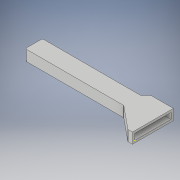
# Autodesk Inventor part: PATAS
Saved by Autodesk Inventor 2019 (Build 230136000, 136)
## iProperties
Created: 2020-12-04
Part Number: PATAS
Material: Generic
Document SubType Name: Modeling
Designer: mihai
Density: 1 g/cm^3
Appearance: Default
Author: mihai
Autodesk Inventor part; units mm, degrees
ref_plane "YZ Plane" through (0, 0, 0) normal (1, 0, 0) x (0, 1, 0)
ref_plane "XZ Plane" through (0, 0, 0) normal (0, 1, 0) x (-1, 0, 0)
ref_plane "XY Plane" through (0, 0, 0) normal (0, 0, 1) x (1, 0, 0)
sketch "Sketch1" plane through (0, 0, 0) normal (0, 1, 0) x (-1, 0, 0)
  line L0 (0, 0) -> (0, -48)
  line L1 (0, 0) -> (4.9, 0)
  line L2 (0, -24) -> (33, -24) construction
  line L3 (0, -48) -> (33, -48) construction
  line L4 (33, -48) -> (33, -43) construction
  line L5 (33, -48) -> (28, -48) construction
  line L6 (0, -48) -> (28, -48)
  line L7 (28, -48) -> (33, -43)
  line L8 (33, -43) -> (33, -23)
  line L9 (4.9, 0) -> (33, -23)
  dimension "d0" = 48
  dimension "d1" = 4.9
  dimension "d2" = 33
  dimension "d3" = 5
  dimension "d4" = 5
  dimension "d5" = 20
  constraints: 20 end point, 3 horizontal, 2 vertical, 1 collinear, 1 midpoint, 1 perpendicular, 1 point on line
  measures "d0" distance of L0.start L0.end
  measures "d1" distance of L0.start L1.end
  measures "d2" distance of L2.start L2.end
  measures "d3" distance of L3.end L4.end
  measures "d4" distance of L3.end L5.end
  measures "d5" distance of L4.end L8.end
extrude "Extrusion1" add sketch "Sketch1" along normal blind 1
sketch "Sketch2" plane through (0, 1, 0) normal (0, 1, 0) x (1, 0, 0)
  line L0 (0, 0) -> (0, 48) projected
  line L1 (0, 48) -> (-28, 48) projected
  line L2 (-28, 48) -> (-33, 43) projected
  line L3 (-33, 43) -> (-33, 23) projected
  line L4 (-33, 23) -> (-4.9, 0) projected
  line L5 (-4.9, 0) -> (0, 0) projected
  line L6 (-5.9712, -3) -> (-36, 21.5787)
  line L7 (-36, 21.5787) -> (-36, 44.2426)
  line L8 (-36, 44.2426) -> (-29.2426, 51)
  line L9 (-29.2426, 51) -> (3, 51)
  line L10 (3, 51) -> (3, -3)
  line L11 (3, -3) -> (-5.9712, -3)
  dimension "d8" = 3
  constraints: 12 end point, 5 other
  measures "d8" distance between parallel lines of L4 L6
extrude "Extrusion2" add sketch "Sketch2" along normal blind 3 contours L5 L4 L3 L2 L1 L0 | L6 L7 L8 L9 L10 L11
sketch "Sketch3" plane through (0, 0, 0) normal (0, -1, 0) x (1, 0, 0)
  line L0 (0, 0) -> (0, -48) projected
  line L1 (-4.9, 0) -> (0, 0) projected
  line L2 (-33, -23) -> (-4.9, 0) projected
  line L3 (-33, -43) -> (-33, -23) projected
  line L4 (-28, -48) -> (-33, -43) projected
  line L5 (0, -48) -> (-28, -48) projected
  line L6 (3, -51) -> (3, 3)
  line L7 (3, 3) -> (-5.9712, 3)
  line L8 (-5.9712, 3) -> (-36, -21.5787)
  line L9 (-36, -21.5787) -> (-36, -44.2426)
  line L10 (-36, -44.2426) -> (-29.2426, -51)
  line L11 (-29.2426, -51) -> (3, -51)
  dimension "d11" = 3
  constraints: 12 end point, 5 other
  measures "d11" distance between parallel lines of L0 L6
extrude "Extrusion3" add sketch "Sketch3" along normal blind 3 contours L0 L5 L4 L3 L2 L1 | L11 L10 L9 L8 L7 L6
sketch "Sketch4" plane through (0, 0, 0) normal (0, 1, 0) x (1, 0, 0)
  line L0 (3, 51) -> (3, -3) projected
  line L1 (-29.2426, 51) -> (3, 51) projected
  line L2 (-36, 44.2426) -> (-29.2426, 51) projected
  line L3 (-36, 21.5787) -> (-36, 44.2426) projected
  line L4 (-5.9712, -3) -> (-36, 21.5787) projected
  line L5 (3, -3) -> (-5.9712, -3) projected
  line L6 (-4.9, 0) -> (0, 0) projected
  line L7 (-33, 23) -> (-4.9, 0) projected
  line L8 (-33, 43) -> (-33, 23) projected
  line L9 (-28, 48) -> (-33, 43) projected
  line L10 (0, 48) -> (-28, 48) projected
  line L11 (0, 0) -> (0, 48) projected
  line L12 (0, 0) -> (0, 48) projected
  line L13 (0, 48) -> (0, 51)
  line L14 (0, 0) -> (0, -3)
  line L15 (3, -3) -> (-5.9712, -3) projected
  constraints: 4 end point, 4 point on line
extrude "Extrusion4" add sketch "Sketch4" along normal blind 8 contours L13 L10 L9 L8 L7 L6 L14 L5 L4 L3 L2 L1
sketch "Sketch5" plane through (-36, 4, -44.2426) normal (-1, 0, 0) x (0, 0, 1)
  line L0 (0, 4) -> (0, -7) projected
  line L1 (22.6639, -7) -> (0, -7) projected
  line L2 (22.6639, 4) -> (22.6639, -7) projected
  line L3 (0, 4) -> (22.6639, 4) projected
  point P0 (44.2426, -4)
extrude "Extrusion5" add sketch "Sketch5" along normal blind 130
fillet "Fillet1" radius 2 6 edges at (-36, 2.5, -44.2426) (-36, 2.5, -21.5787) (-5.9712, 2.5, 3) (-29.2426, 2.5, -51) (-166, 2.5, -44.2426) (-166, 2.5, -21.5787)
sketch "Sketch6" plane through (0, 0, 0) normal (0, 1, 0) x (1, 0, 0)
  line L0 (0, -3) -> (0, 51) projected
  line L1 (3, -3) -> (0, -3) projected
  line L2 (3, 51) -> (3, -3) projected
  line L3 (0, 51) -> (3, 51) projected
  point P0 (0, 0)
extrude "Extrusion6" cut sketch "Sketch6" along normal blind 130 and the other way blind 65
sketch "Sketch7" plane through (0, 4, 0) normal (0, 1, 0) x (1, 0, 0)
  line L0 (0, 0) -> (0, 48) projected
  line L1 (0, 48) -> (-28, 48) projected
  line L2 (-28, 48) -> (-33, 43) projected
  line L3 (-33, 43) -> (-33, 23) projected
  line L4 (-33, 23) -> (-4.9, 0) projected
  line L5 (-4.9, 0) -> (0, 0) projected
extrude "Extrusion7" cut sketch "Sketch7" against normal blind 4
sketch "Sketch8" plane through (0, -3, 3) normal (1, 0, 0) x (0, 0, -1)
  point P0 (3, 3)
sketch "Sketch9" plane through (0, 8, 0) normal (0, 1, 0) x (1, 0, 0)
  line L0 (0, 48) -> (0, 0) projected
  line L1 (-28, 48) -> (0, 48) projected
  line L2 (-33, 43) -> (-28, 48) projected
  line L3 (-33, 23) -> (-33, 43) projected
  line L4 (-4.9, 0) -> (-33, 23) projected
  line L5 (0, 0) -> (-4.9, 0) projected
  arc A0 (-166, 23.5787) -> (-164, 21.5787) centre (-164, 23.5787) ccw projected
  line L6 (-36.7141, 21.5787) -> (-164, 21.5787) projected
  arc A1 (-35.4474, 21.1264) -> (-36.7141, 21.5787) centre (-36.7141, 19.5787) ccw projected
  line L7 (-35.4474, 21.1264) -> (-6.5238, -2.5477) projected
  arc A2 (-6.5238, -2.5477) -> (-5.2571, -3) centre (-5.2571, -1) ccw projected
  line L8 (-5.2571, -3) -> (0, -3) projected
  line L9 (0, -3) -> (0, 0) projected
  line L10 (0, 0) -> (-4.9, 0) projected
  line L11 (-4.9, 0) -> (-33, 23) projected
  line L12 (-33, 23) -> (-33, 43) projected
  line L13 (-33, 43) -> (-28, 48) projected
  line L14 (-28, 48) -> (0, 48) projected
  line L15 (0, 48) -> (0, 51) projected
  line L16 (0, 51) -> (-28.4142, 51) projected
  arc A3 (-28.4142, 51) -> (-29.8284, 50.4142) centre (-28.4142, 49) ccw projected
  line L17 (-29.8284, 50.4142) -> (-35.4142, 44.8284) projected
  arc A4 (-36.8284, 44.2426) -> (-35.4142, 44.8284) centre (-36.8284, 46.2426) ccw projected
  line L18 (-36.8284, 44.2426) -> (-164, 44.2426) projected
  arc A5 (-164, 44.2426) -> (-166, 42.2426) centre (-164, 42.2426) ccw projected
  line L19 (-166, 23.5787) -> (-166, 42.2426) projected
extrude "Extrusion8" add sketch "Sketch9" along normal blind 3
body "Solid1"
